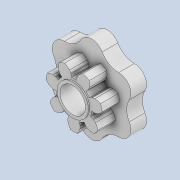
# Autodesk Inventor part: m1z7
Saved by Autodesk Inventor 2020.4 (Build 244396000, 396)
## iProperties
Created: 2021-04-23
Part Number: m1z7
Material: アルミニウム 2014-T4
Document SubType Name: Modeling
Designer: happy
Density: 2.8 g/cm^3
Appearance: サテン
Author: happy
Autodesk Inventor part; units mm, degrees
ref_plane "YZ Plane" through (0, 0, 0) normal (1, 0, 0) x (0, 1, 0)
ref_plane "XZ Plane" through (0, 0, 0) normal (0, 1, 0) x (-1, 0, 0)
ref_plane "XY Plane" through (0, 0, 0) normal (0, 0, 1) x (1, 0, 0)
sketch "スケッチ1" plane through (0, 0, 0) normal (0, 0, 1) x (1, 0, 0)
  arc A0 (149.0124, 108.3484) -> (148.9774, 108.2273) centre (149.4432, 108.1583) ccw
  arc A1 (149.2206, 108.6783) -> (149.0124, 108.3484) centre (150.2273, 107.8124) ccw
  arc A2 (149.9571, 109.2576) -> (149.2206, 108.6783) centre (151.0635, 107.0931) ccw
  arc A3 (146.2017, 107.4883) -> (146.2745, 107.3855) centre (146.6188, 107.7066) ccw
  arc A4 (146.0735, 107.8567) -> (146.2017, 107.4883) centre (147.3782, 108.104) ccw
  arc A5 (146.0798, 108.7937) -> (146.0735, 107.8567) centre (148.4618, 108.3094) ccw
  arc A6 (145.1216, 104.7545) -> (145.2474, 104.7474) centre (145.211, 105.2168) ccw
  arc A7 (144.7536, 104.8841) -> (145.1216, 104.7545) centre (145.3738, 106.0583) ccw
  arc A8 (144.0249, 105.4731) -> (144.7536, 104.8841) centre (145.8888, 107.0335) ccw
  arc A9 (146.5855, 102.2056) -> (146.6695, 102.2995) centre (146.2798, 102.5637) ccw
  arc A10 (146.2548, 101.9987) -> (146.5855, 102.2056) centre (145.7234, 103.2156) ccw
  arc A11 (145.3399, 101.7963) -> (146.2548, 101.9987) centre (145.2821, 104.2264) ccw
  arc A12 (149.4911, 101.7609) -> (149.4701, 101.8851) centre (149.0205, 101.7452) ccw
  arc A13 (149.4467, 101.3734) -> (149.4911, 101.7609) centre (148.1639, 101.7167) ccw
  arc A14 (149.0345, 100.5319) -> (149.4467, 101.3734) centre (147.0985, 102.0018) ccw
  arc A15 (151.6504, 103.7553) -> (151.5401, 103.8163) centre (151.3692, 103.3776) ccw
  arc A16 (151.9257, 103.479) -> (151.6504, 103.7553) centre (150.8575, 102.6901) ccw
  arc A17 (152.3266, 102.6321) -> (151.9257, 103.479) centre (149.9703, 102.0349) ccw
  arc A18 (151.4374, 106.687) -> (151.3209, 106.6389) centre (151.5574, 106.2317) ccw
  arc A19 (151.8251, 106.7299) -> (151.4374, 106.687) centre (151.7758, 105.4029) ccw
  arc A20 (152.7372, 106.5154) -> (151.8251, 106.7299) centre (151.7349, 104.3008) ccw
  arc A21 (148.0225, 108.2273) -> (147.9875, 108.3483) centre (147.5568, 108.1583) ccw
  arc A22 (147.9875, 108.3483) -> (147.7794, 108.6782) centre (146.7726, 107.8124) ccw
  arc A23 (147.7794, 108.6782) -> (147.0429, 109.2576) centre (145.9364, 107.0932) ccw
  arc A24 (145.6791, 106.6389) -> (145.5626, 106.687) centre (145.4426, 106.2317) ccw
  arc A25 (145.5626, 106.687) -> (145.1749, 106.7299) centre (145.2242, 105.4029) ccw
  arc A26 (145.1749, 106.7299) -> (144.2628, 106.5154) centre (145.2651, 104.3008) ccw
  arc A27 (145.4599, 103.8163) -> (145.3496, 103.7553) centre (145.6308, 103.3776) ccw
  arc A28 (145.3496, 103.7553) -> (145.0743, 103.479) centre (146.1425, 102.6901) ccw
  arc A29 (145.0743, 103.479) -> (144.6734, 102.6321) centre (147.0297, 102.0349) ccw
  arc A30 (147.5299, 101.8851) -> (147.5089, 101.7609) centre (147.9795, 101.7452) ccw
  arc A31 (147.5089, 101.7609) -> (147.5533, 101.3734) centre (148.8361, 101.7167) ccw
  arc A32 (147.5533, 101.3734) -> (147.9655, 100.5319) centre (149.9015, 102.0018) ccw
  arc A33 (150.3305, 102.2995) -> (150.4145, 102.2056) centre (150.7202, 102.5637) ccw
  arc A34 (150.4145, 102.2056) -> (150.7452, 101.9987) centre (151.2766, 103.2156) ccw
  arc A35 (150.7452, 101.9987) -> (151.6601, 101.7963) centre (151.7179, 104.2264) ccw
  arc A36 (151.7526, 104.7474) -> (151.8784, 104.7545) centre (151.789, 105.2168) ccw
  arc A37 (151.8784, 104.7545) -> (152.2464, 104.8841) centre (151.6262, 106.0583) ccw
  arc A38 (152.2464, 104.8841) -> (152.9751, 105.4731) centre (151.1112, 107.0335) ccw
  arc A39 (150.7255, 107.3855) -> (150.7983, 107.4883) centre (150.3812, 107.7066) ccw
  arc A40 (150.7983, 107.4883) -> (150.9265, 107.8567) centre (149.6218, 108.104) ccw
  arc A41 (150.9265, 107.8567) -> (150.9202, 108.7937) centre (148.5382, 108.3094) ccw
  arc A42 (148.917, 107.8193) -> (148.083, 107.8193) centre (148.5, 105) ccw
  arc A43 (146.5558, 107.0839) -> (146.0358, 106.4318) centre (148.5, 105) ccw
  arc A44 (145.6586, 104.7792) -> (145.8442, 103.9661) centre (148.5, 105) ccw
  arc A45 (146.901, 102.6408) -> (147.6525, 102.2789) centre (148.5, 105) ccw
  arc A46 (149.3475, 102.2789) -> (150.099, 102.6408) centre (148.5, 105) ccw
  arc A47 (151.1558, 103.9661) -> (151.3414, 104.7792) centre (148.5, 105) ccw
  arc A48 (150.9642, 106.4318) -> (150.4442, 107.0839) centre (148.5, 105) ccw
  arc A49 (147.0429, 109.2576) -> (146.0798, 108.7937) centre (148.5, 105) ccw
  arc A50 (144.2628, 106.5154) -> (144.0249, 105.4731) centre (148.5, 105) ccw
  arc A51 (144.6734, 102.6321) -> (145.3399, 101.7963) centre (148.5, 105) ccw
  arc A52 (147.9655, 100.5319) -> (149.0345, 100.5319) centre (148.5, 105) ccw
  arc A53 (151.6601, 101.7963) -> (152.3266, 102.6321) centre (148.5, 105) ccw
  arc A54 (152.9751, 105.4731) -> (152.7372, 106.5154) centre (148.5, 105) ccw
  arc A55 (150.9202, 108.7937) -> (149.9571, 109.2576) centre (148.5, 105) ccw
  line L0 (148.917, 107.8193) -> (148.9774, 108.2273)
  line L1 (146.5558, 107.0839) -> (146.2745, 107.3855)
  line L2 (145.6586, 104.7792) -> (145.2474, 104.7474)
  line L3 (146.901, 102.6408) -> (146.6695, 102.2995)
  line L4 (149.3475, 102.2789) -> (149.4701, 101.8851)
  line L5 (151.1558, 103.9661) -> (151.5401, 103.8163)
  line L6 (150.9642, 106.4318) -> (151.3209, 106.6389)
  line L7 (148.083, 107.8193) -> (148.0225, 108.2273)
  line L8 (146.0358, 106.4318) -> (145.6791, 106.6389)
  line L9 (145.8442, 103.9661) -> (145.4599, 103.8163)
  line L10 (147.6525, 102.2789) -> (147.5299, 101.8851)
  line L11 (150.099, 102.6408) -> (150.3305, 102.2995)
  line L12 (151.3414, 104.7792) -> (151.7526, 104.7474)
  line L13 (150.4442, 107.0839) -> (150.7255, 107.3855)
  line L14 (142, 105) -> (155, 105)
  line L15 (148.5, 98.5) -> (148.5, 111.5)
  line L16 (173, 109.5) -> (243, 109.5)
  line L17 (173, 101.5) -> (243, 101.5)
  line L18 (173, 93.5) -> (243, 93.5)
  line L19 (173, 85.5) -> (243, 85.5)
  line L20 (173, 77.5) -> (243, 77.5)
  line L21 (173, 69.5) -> (243, 69.5)
  line L22 (173, 61.5) -> (243, 61.5)
  line L23 (173, 53.5) -> (243, 53.5)
  line L24 (173, 45.5) -> (243, 45.5)
  line L25 (173, 37.5) -> (243, 37.5)
  line L26 (173, 29.5) -> (243, 29.5)
  line L27 (173, 21.5) -> (243, 21.5)
  line L28 (173, 13.5) -> (243, 13.5)
  line L29 (173, 109.5) -> (173, 13.5)
  line L30 (243, 109.5) -> (243, 13.5)
  line L31 (208, 101.5) -> (208, 13.5)
  circle A56 centre (148.5, 105) radius 8
  circle A57 centre (148.5, 105) radius 7 construction
  line L32 (148.5, 112) -> (154.5622, 108.5) construction
  line L33 (154.5622, 108.5) -> (154.5622, 101.5) construction
  line L34 (154.5622, 101.5) -> (148.5, 98) construction
  line L35 (148.5, 98) -> (142.4378, 101.5) construction
  line L36 (142.4378, 108.5) -> (148.5, 112) construction
  arc A58 (150.2321, 111) -> (146.7679, 111) centre (148.5, 110) ccw
  arc A59 (144.1699, 109.5) -> (142.4378, 106.5) centre (144.1699, 107.5) ccw
  arc A60 (142.4378, 103.5) -> (144.1699, 100.5) centre (144.1699, 102.5) ccw
  arc A61 (146.7679, 99) -> (150.2321, 99) centre (148.5, 100) ccw
  arc A62 (152.8301, 100.5) -> (154.5622, 103.5) centre (152.8301, 102.5) ccw
  arc A63 (154.5622, 106.5) -> (152.8301, 109.5) centre (152.8301, 107.5) ccw
  arc A64 (150.2321, 111) -> (152.8301, 109.5) centre (152.8301, 112.5) ccw
  arc A65 (144.1699, 109.5) -> (146.7679, 111) centre (144.1699, 112.5) ccw
  arc A66 (142.4378, 103.5) -> (142.4378, 106.5) centre (139.8397, 105) ccw
  arc A67 (146.7679, 99) -> (144.1699, 100.5) centre (144.1699, 97.5) ccw
  arc A68 (152.8301, 100.5) -> (150.2321, 99) centre (152.8301, 97.5) ccw
  arc A69 (154.5622, 106.5) -> (154.5622, 103.5) centre (157.1603, 105) ccw
  circle A70 centre (148.5, 105) radius 5.6603 construction
  circle A71 centre (148.5, 105) radius 2.025
  point P0 (0, 0)
  point P1 (179, 103.5)
  point P2 (181.5, 95.5)
  point P3 (181.5, 87.5)
  point P4 (179, 79.5)
  point P5 (181.5, 71.5)
  point P6 (176.5, 63.5)
  point P7 (179, 55.5)
  point P8 (179, 47.5)
  point P9 (179, 39.5)
  point P10 (181.5, 31.5)
  point P11 (181.5, 23.5)
  point P12 (179, 15.5)
  point P13 (209, 95.5)
  point P14 (225.25, 87.5)
  point P15 (225.25, 79.5)
  point P16 (221.5, 71.5)
  point P17 (225.25, 63.5)
  point P18 (219, 55.5)
  point P19 (225.25, 47.5)
  point P20 (222.75, 39.5)
  point P21 (219, 31.5)
  point P22 (226.5, 23.5)
  point P23 (226.5, 15.5)
  point P24 (149.5, 125)
  point P25 (149.5, 119)
  point P26 (167.8125, 125)
  point P27 (168.875, 119)
  point P28 (142.4378, 108.5)
  point P29 (142.4378, 101.5)
  point P30 (148.5, 98)
  point P31 (154.5622, 101.5)
  point P32 (154.5622, 108.5)
  point P33 (154.5622, 106.5)
  point P34 (142.4378, 103.5)
  point P35 (144.1699, 100.5)
  point P36 (146.7679, 99)
  dimension "d5" = 14
  dimension "d4" = 16
  dimension "d6" = 360
  dimension "d7" = 360
  dimension "d8" = 11.3205
  dimension "d9" = 3
  dimension "d10" = 2
  dimension "d15" = 4.05
  constraints: 142 point on circle, 71 centre point, 70 end point, 51 tangent, 39 equal radius, 13 parallel, 6 concentric, 5 coincident, 3 horizontal, 3 midpoint, 2 perpendicular, 2 point on line, 2 vertical, 1 vertical alignment, 312 other
  measures "d4" diameter of A56
  measures "d8" diameter of A70
  measures "d9" radius of A64
  measures "d10" radius of A58
  measures "d15" diameter of A71
extrude "押し出し1" add sketch "スケッチ1" along normal blind 2.8 contours A1 A2 A55 A41 A40 A39 L13 A48 L6 A18 A19 A20 A54 A38 L14 A71 L15 A42 L0 A0 | L15 A71 L14 A8 A50 A26 A25 A24 L8 A43 L1 A3 A4 A5 A49 A23 A22 A21 L7 A42 | L14 A38 A37 A36 L12 A47 L5 A15 A16 A17 A53 A35 A34 A33 L11 A46 L4 A12 A13 A14 A52 L15 A71 | A71 L15 A52 A32 A31 A30 L10 A45 L3 A9 A10 A11 A51 A29 A28 A27 L9 A44 L2 A6 A7 A8 L14
extrude "押し出し2" add sketch "スケッチ1" against normal blind 2.5 contours A1 A2 A55 A41 A40 A39 L13 A48 L6 A18 A19 A20 A54 A38 L14 A71 L15 A42 L0 A0 | A0 L0 A42 L7 A21 A22 A23 A49 A5 A4 A3 L1 A43 L8 A24 A25 A26 A50 A8 L14 A66 A59 A65 A58 A64 A63 A69 A38 A54 A20 A19 A18 L6 A48 L13 A39 A40 A41 A55 A2 A1 | L15 A71 L14 A8 A50 A26 A25 A24 L8 A43 L1 A3 A4 A5 A49 A23 A22 A21 L7 A42 | L14 A38 A37 A36 L12 A47 L5 A15 A16 A17 A53 A35 A34 A33 L11 A46 L4 A12 A13 A14 A52 L15 A71 | A71 L15 A52 A32 A31 A30 L10 A45 L3 A9 A10 A11 A51 A29 A28 A27 L9 A44 L2 A6 A7 A8 L14 | L14 A69 A62 A68 A61 A67 A60 A66 A8 A7 A6 L2 A44 L9 A27 A28 A29 A51 A11 A10 A9 L3 A45 L10 A30 A31 A32 A52 A14 A13 A12 L4 A46 L11 A33 A34 A35 A53 A17 A16 A15 L5 A47 L12 A36 A37 A38
sketch "スケッチ2" plane through (0, 0, 2.8) normal (0, 0, 1) x (1, 0, 0)
  line L0 (148.083, 107.8193) -> (148.0225, 108.2273) projected
  arc A0 (148.0225, 108.2273) -> (147.9875, 108.3483) centre (147.5568, 108.1583) ccw projected
  arc A1 (147.9875, 108.3483) -> (147.7794, 108.6782) centre (146.7726, 107.8124) ccw projected
  arc A2 (147.7794, 108.6782) -> (147.0429, 109.2576) centre (145.9364, 107.0932) ccw projected
  arc A3 (147.0429, 109.2576) -> (146.0798, 108.7937) centre (148.5, 105) ccw projected
  arc A4 (146.0798, 108.7937) -> (146.0735, 107.8567) centre (148.4618, 108.3094) ccw projected
  arc A5 (146.0735, 107.8567) -> (146.2017, 107.4883) centre (147.3782, 108.104) ccw projected
  arc A6 (146.2017, 107.4883) -> (146.2745, 107.3855) centre (146.6188, 107.7066) ccw projected
  line L1 (146.2745, 107.3855) -> (146.5558, 107.0839) projected
  arc A7 (146.5558, 107.0839) -> (146.0358, 106.4318) centre (148.5, 105) ccw projected
  line L2 (146.0358, 106.4318) -> (145.6791, 106.6389) projected
  arc A8 (145.6791, 106.6389) -> (145.5626, 106.687) centre (145.4426, 106.2317) ccw projected
  arc A9 (145.5626, 106.687) -> (145.1749, 106.7299) centre (145.2242, 105.4029) ccw projected
  arc A10 (145.1749, 106.7299) -> (144.2628, 106.5154) centre (145.2651, 104.3008) ccw projected
  arc A11 (144.2628, 106.5154) -> (144.0249, 105.4731) centre (148.5, 105) ccw projected
  arc A12 (144.0249, 105.4731) -> (144.7536, 104.8841) centre (145.8888, 107.0335) ccw projected
  arc A13 (144.7536, 104.8841) -> (145.1216, 104.7545) centre (145.3738, 106.0583) ccw projected
  arc A14 (145.1216, 104.7545) -> (145.2474, 104.7474) centre (145.211, 105.2168) ccw projected
  line L3 (145.2474, 104.7474) -> (145.6586, 104.7792) projected
  arc A15 (145.6586, 104.7792) -> (145.8442, 103.9661) centre (148.5, 105) ccw projected
  line L4 (145.8442, 103.9661) -> (145.4599, 103.8163) projected
  arc A16 (145.4599, 103.8163) -> (145.3496, 103.7553) centre (145.6308, 103.3776) ccw projected
  arc A17 (145.3496, 103.7553) -> (145.0743, 103.479) centre (146.1425, 102.6901) ccw projected
  arc A18 (145.0743, 103.479) -> (144.6734, 102.6321) centre (147.0297, 102.0349) ccw projected
  arc A19 (144.6734, 102.6321) -> (145.3399, 101.7963) centre (148.5, 105) ccw projected
  arc A20 (145.3399, 101.7963) -> (146.2548, 101.9987) centre (145.2821, 104.2264) ccw projected
  arc A21 (146.2548, 101.9987) -> (146.5855, 102.2056) centre (145.7234, 103.2156) ccw projected
  arc A22 (146.5855, 102.2056) -> (146.6695, 102.2995) centre (146.2798, 102.5637) ccw projected
  line L5 (146.6695, 102.2995) -> (146.901, 102.6408) projected
  arc A23 (146.901, 102.6408) -> (147.6525, 102.2789) centre (148.5, 105) ccw projected
  line L6 (147.6525, 102.2789) -> (147.5299, 101.8851) projected
  arc A24 (147.5299, 101.8851) -> (147.5089, 101.7609) centre (147.9795, 101.7452) ccw projected
  arc A25 (147.5089, 101.7609) -> (147.5533, 101.3734) centre (148.8361, 101.7167) ccw projected
  arc A26 (147.5533, 101.3734) -> (147.9655, 100.5319) centre (149.9015, 102.0018) ccw projected
  arc A27 (147.9655, 100.5319) -> (149.0345, 100.5319) centre (148.5, 105) ccw projected
  arc A28 (149.0345, 100.5319) -> (149.4467, 101.3734) centre (147.0985, 102.0018) ccw projected
  arc A29 (149.4467, 101.3734) -> (149.4911, 101.7609) centre (148.1639, 101.7167) ccw projected
  arc A30 (149.4911, 101.7609) -> (149.4701, 101.8851) centre (149.0205, 101.7452) ccw projected
  line L7 (149.4701, 101.8851) -> (149.3475, 102.2789) projected
  arc A31 (149.3475, 102.2789) -> (150.099, 102.6408) centre (148.5, 105) ccw projected
  line L8 (150.099, 102.6408) -> (150.3305, 102.2995) projected
  arc A32 (150.3305, 102.2995) -> (150.4145, 102.2056) centre (150.7202, 102.5637) ccw projected
  arc A33 (150.4145, 102.2056) -> (150.7452, 101.9987) centre (151.2766, 103.2156) ccw projected
  arc A34 (150.7452, 101.9987) -> (151.6601, 101.7963) centre (151.7179, 104.2264) ccw projected
  arc A35 (151.6601, 101.7963) -> (152.3266, 102.6321) centre (148.5, 105) ccw projected
  arc A36 (152.3266, 102.6321) -> (151.9257, 103.479) centre (149.9703, 102.0349) ccw projected
  arc A37 (151.9257, 103.479) -> (151.6504, 103.7553) centre (150.8575, 102.6901) ccw projected
  arc A38 (151.6504, 103.7553) -> (151.5401, 103.8163) centre (151.3692, 103.3776) ccw projected
  line L9 (151.5401, 103.8163) -> (151.1558, 103.9661) projected
  arc A39 (151.1558, 103.9661) -> (151.3414, 104.7792) centre (148.5, 105) ccw projected
  line L10 (151.3414, 104.7792) -> (151.7526, 104.7474) projected
  arc A40 (151.7526, 104.7474) -> (151.8784, 104.7545) centre (151.789, 105.2168) ccw projected
  arc A41 (151.8784, 104.7545) -> (152.2464, 104.8841) centre (151.6262, 106.0583) ccw projected
  arc A42 (152.2464, 104.8841) -> (152.9751, 105.4731) centre (151.1112, 107.0335) ccw projected
  arc A43 (152.9751, 105.4731) -> (152.7372, 106.5154) centre (148.5, 105) ccw projected
  arc A44 (152.7372, 106.5154) -> (151.8251, 106.7299) centre (151.7349, 104.3008) ccw projected
  arc A45 (151.8251, 106.7299) -> (151.4374, 106.687) centre (151.7758, 105.4029) ccw projected
  arc A46 (151.4374, 106.687) -> (151.3209, 106.6389) centre (151.5574, 106.2317) ccw projected
  line L11 (151.3209, 106.6389) -> (150.9642, 106.4318) projected
  arc A47 (150.9642, 106.4318) -> (150.4442, 107.0839) centre (148.5, 105) ccw projected
  line L12 (150.4442, 107.0839) -> (150.7255, 107.3855) projected
  arc A48 (150.7255, 107.3855) -> (150.7983, 107.4883) centre (150.3812, 107.7066) ccw projected
  arc A49 (150.7983, 107.4883) -> (150.9265, 107.8567) centre (149.6218, 108.104) ccw projected
  arc A50 (150.9265, 107.8567) -> (150.9202, 108.7937) centre (148.5382, 108.3094) ccw projected
  arc A51 (150.9202, 108.7937) -> (149.9571, 109.2576) centre (148.5, 105) ccw projected
  arc A52 (149.9571, 109.2576) -> (149.2206, 108.6783) centre (151.0635, 107.0931) ccw projected
  arc A53 (149.2206, 108.6783) -> (149.0124, 108.3484) centre (150.2273, 107.8124) ccw projected
  arc A54 (149.0124, 108.3484) -> (148.9774, 108.2273) centre (149.4432, 108.1583) ccw projected
  line L13 (148.9774, 108.2273) -> (148.917, 107.8193) projected
  arc A55 (148.917, 107.8193) -> (148.083, 107.8193) centre (148.5, 105) ccw projected
  circle A56 centre (148.5, 105) radius 2.025 projected
  circle A57 centre (148.5, 105) radius 2.025 projected
  circle A58 centre (148.5, 105) radius 2.5
  point P0 (0, 0)
  dimension "d16" = 5
  constraints: 1 centre point, 1 coincident
  measures "d16" diameter of A58
extrude "押し出し3" add sketch "スケッチ2" along normal blind 0.2 contours A58
sketch "スケッチ3" plane through (0, 0, -2.5) normal (0, 0, -1) x (-1, 0, 0)
  arc A0 (-152.8301, 109.5) -> (-154.5622, 106.5) centre (-152.8301, 107.5) ccw projected
  arc A1 (-154.5622, 103.5) -> (-154.5622, 106.5) centre (-157.1603, 105) ccw projected
  arc A2 (-154.5622, 103.5) -> (-152.8301, 100.5) centre (-152.8301, 102.5) ccw projected
  arc A3 (-150.2321, 99) -> (-152.8301, 100.5) centre (-152.8301, 97.5) ccw projected
  arc A4 (-150.2321, 99) -> (-146.7679, 99) centre (-148.5, 100) ccw projected
  arc A5 (-144.1699, 100.5) -> (-146.7679, 99) centre (-144.1699, 97.5) ccw projected
  arc A6 (-144.1699, 100.5) -> (-142.4378, 103.5) centre (-144.1699, 102.5) ccw projected
  arc A7 (-142.4378, 106.5) -> (-142.4378, 103.5) centre (-139.8397, 105) ccw projected
  arc A8 (-142.4378, 106.5) -> (-144.1699, 109.5) centre (-144.1699, 107.5) ccw projected
  arc A9 (-146.7679, 111) -> (-144.1699, 109.5) centre (-144.1699, 112.5) ccw projected
  arc A10 (-146.7679, 111) -> (-150.2321, 111) centre (-148.5, 110) ccw projected
  arc A11 (-152.8301, 109.5) -> (-150.2321, 111) centre (-152.8301, 112.5) ccw projected
  circle A12 centre (-148.5, 105) radius 2.025 projected
  arc A13 (-142.4811, 106.525) -> (-144.1699, 109.45) centre (-144.1699, 107.5) ccw
  arc A14 (-142.4811, 106.525) -> (-142.4811, 103.475) centre (-139.8397, 105) ccw
  arc A15 (-144.1699, 100.55) -> (-142.4811, 103.475) centre (-144.1699, 102.5) ccw
  arc A16 (-144.1699, 100.55) -> (-146.8113, 99.025) centre (-144.1699, 97.5) ccw
  arc A17 (-150.1887, 99.025) -> (-146.8113, 99.025) centre (-148.5, 100) ccw
  arc A18 (-150.1887, 99.025) -> (-152.8301, 100.55) centre (-152.8301, 97.5) ccw
  arc A19 (-154.5189, 103.475) -> (-152.8301, 100.55) centre (-152.8301, 102.5) ccw
  arc A20 (-154.5189, 103.475) -> (-154.5189, 106.525) centre (-157.1603, 105) ccw
  arc A21 (-152.8301, 109.45) -> (-154.5189, 106.525) centre (-152.8301, 107.5) ccw
  arc A22 (-152.8301, 109.45) -> (-150.1887, 110.975) centre (-152.8301, 112.5) ccw
  arc A23 (-146.8113, 110.975) -> (-150.1887, 110.975) centre (-148.5, 110) ccw
  arc A24 (-146.8113, 110.975) -> (-144.1699, 109.45) centre (-144.1699, 112.5) ccw
  point P0 (0, 0)
  dimension "d19" = 0.05
  constraints: 24 point on circle, 12 centre point, 11 other
  measures "d19" radial gap between concentric circles of A8 A13
extrude "押し出し4" cut sketch "スケッチ3" against normal blind 10 contours A11 A10 A9 A8 A7 A6 A5 A4 A3 A2 A1 A0
